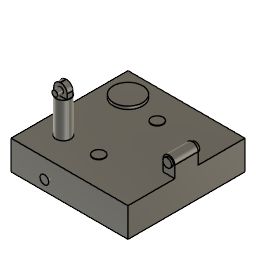
Soil Detector Rover (Autodesk Fusion 360 archive; units mm, degrees)
design "base"
part number: 2026-08-26-18-15-48-406
Autodesk Fusion 360 part; units mm, degrees
sketch "Sketch1" plane through (0, 0, 0) normal (0, 0, 1) x (1, 0, 0)
  line L0 (100, 100) -> (-100, 100)
  line L1 (-100, 100) -> (-100, -100)
  line L2 (-100, -100) -> (100, -100)
  line L3 (100, -100) -> (100, 100)
  line L4 (100, 100) -> (-100, -100) construction
  line L5 (-100, 100) -> (100, -100) construction
  dimension "d1" = 200
  dimension "d2" = 200
  constraint horizontal L0
  constraint perpendicular L0 L1
  constraint parallel L0 L2
  constraint parallel L1 L3
  constraint coincident L4 origin
  constraint coincident L5 origin
  measures "d1" distance of L0.end L1.end
  measures "d2" distance of L0.start L0.end
extrude "Extrude1" add sketch "Sketch1" along normal blind 50 makes body 1
sketch "Sketch2" plane through (0, 0, 50) normal (0, 0, 1) x (-1, 0, 0)
  line L0 (-100, 100) -> (-100, -100)
  line L1 (-100, -100) -> (100, -100)
  line L2 (100, -100) -> (100, 100)
  line L3 (100, 100) -> (-100, 100)
  circle A0 centre (60, 50.4709) radius 12.5
  dimension "d5" = 25
  dimension "d6" = 40
  measures "d5" diameter of A0
  measures "d6" distance of L2 A0.centre
extrude "Extrude2" add sketch "Sketch2" along normal blind 60 contours A0 bodies 1
sketch "Sketch3" plane through (0, 0, 110) normal (0, 0, 1) x (-1, 0, 0)
  circle A0 centre (60, 50.4709) radius 12.5
  line L0 (71.4564, 55.4709) -> (48.5436, 55.4709)
  line L1 (48.5436, 55.4709) -> (48.5436, 45.4709)
  line L2 (48.5436, 45.4709) -> (71.4564, 45.4709)
  line L3 (71.4564, 45.4709) -> (71.4564, 55.4709)
  line L4 (71.4564, 55.4709) -> (48.5436, 45.4709) construction
  line L5 (48.5436, 55.4709) -> (71.4564, 45.4709) construction
  circle A1 centre (60, 50.4709) radius 12.5
  point P0 (60, 50.4709)
  dimension "d10" = 10
  constraint horizontal L0
  constraint perpendicular L0 L1
  constraint parallel L0 L2
  constraint parallel L1 L3
  constraint coincident L4 P0
  constraint coincident L5 P0
  constraint coincident P0 A0.centre
  constraint coincident L1.end A1
  measures "d10" distance of L0.end L1.end
extrude "Extrude3" add sketch "Sketch3" along normal blind 20 contours L0 L1 L2 L3 bodies 1
fillet "Fillet1" radius 11.3 2 edges at (-71.4564, -50.4709, 130) (-48.5436, -50.4709, 130) on bodies 1
sketch "Sketch4" plane through (0, -55.4709, 0) normal (0, -1, 0) x (1, 0, 0)
  arc A0 (-48.5436, 118.7) -> (-59.8436, 130) centre (-59.8436, 118.7) ccw
  line L0 (-59.8436, 130) -> (-60.1564, 130)
  arc A1 (-60.1564, 130) -> (-71.4564, 118.7) centre (-60.1564, 118.7) ccw
  line L1 (-71.4564, 118.7) -> (-71.4564, 110)
  line L2 (-71.4564, 110) -> (-48.5436, 110)
  line L3 (-48.5436, 110) -> (-48.5436, 118.7)
  circle A2 centre (-59.8436, 118.7) radius 5
  dimension "d18" = 10
  constraint concentric A0 A2
  measures "d18" diameter of A2
extrude "Extrude4" add sketch "Sketch4" along normal blind 10 contours A2 bodies 1
sketch "Sketch5" plane through (0, 0, 50) normal (0, 0, 1) x (-1, 0, 0)
  circle A0 centre (60, 50.4709) radius 12.5
  line L0 (-100, 100) -> (-100, -100)
  line L1 (-100, -100) -> (100, -100)
  line L2 (100, -100) -> (100, 100)
  line L3 (100, 100) -> (-100, 100)
  line L4 (100, -60) -> (0, -60) construction
  line L5 (60, -100) -> (60, 0) construction
  circle A1 centre (60, -60) radius 25
  dimension "d21" = 50
  constraint coincident L2 L4.start
  constraint perpendicular L2 L4
  constraint coincident L1 L5.start
  constraint perpendicular L4 L5
  constraint coincident L4 A1.centre
  constraint coincident L5 A1.centre
  measures "d21" diameter of A1
extrude "Extrude5" add sketch "Sketch5" along normal blind 5 contours A1 bodies 1
sketch "Sketch6" plane through (0, -100, 0) normal (0, -1, 0) x (1, 0, 0)
  line L0 (-100, 0) -> (100, 0)
  line L1 (100, 0) -> (100, 50)
  line L2 (100, 50) -> (-100, 50)
  line L3 (-100, 50) -> (-100, 0)
  circle A0 centre (-40, 20) radius 7.5
  dimension "d24" = 15
  dimension "d25" = 60
  dimension "d26" = 20
  measures "d24" diameter of A0
  measures "d25" distance of L3 A0.centre
  measures "d26" distance of L0 A0.centre
extrude "Extrude6" add sketch "Sketch6" along normal blind 3 and the other way blind 203 separate body contours A0 makes body 2
sketch "Sketch7" plane through (0, 0, 50) normal (0, 0, 1) x (-1, 0, 0)
  circle A0 centre (60, -60) radius 25
  circle A1 centre (60, 50.4709) radius 12.5
  line L0 (-100, 100) -> (-100, -100)
  line L1 (-100, -100) -> (100, -100)
  line L2 (100, -100) -> (100, 100)
  line L3 (100, 100) -> (-100, 100)
  line L4 (-100, -20) -> (-80, -20)
  line L5 (-80, -20) -> (-80, 20)
  line L6 (-80, 20) -> (-100, 20)
  line L7 (-100, 20) -> (-100, -20)
  dimension "d31" = 20
  dimension "d32" = 40
  constraint horizontal L4
  constraint vertical L5
  constraint horizontal L6
  constraint vertical L7
  constraint coincident L0 L4.start
  measures "d31" distance of L4.start L4.end
  measures "d32" distance of L4.end L5.end
extrude "Extrude7" add sketch "Sketch7" along normal blind 30 contours L0 L4 L5 L6 L7 bodies 1
fillet "Fillet2" radius 10 2 edges at (100, 0, 80) (80, 0, 80) on bodies 1
sketch "Sketch8" plane through (0, -20, 0) normal (0, -1, 0) x (1, 0, 0)
  arc A0 (100, 70) -> (80, 70) centre (90, 70) ccw
  line L0 (80, 70) -> (80, 50)
  line L1 (80, 50) -> (100, 50)
  line L2 (100, 50) -> (100, 70)
  circle A1 centre (90, 70) radius 7.5
  dimension "d37" = 15
  constraint concentric A0 A1
  measures "d37" diameter of A1
extrude "Extrude8" add sketch "Sketch8" along normal blind 3 contours A1 bodies 1
sketch "Sketch9" plane through (0, 0, 50) normal (0, 0, 1) x (-1, 0, 0)
  line L0 (-80, -20) -> (-100, -20)
  line L1 (-100, -20) -> (-100, -100)
  line L2 (-100, -100) -> (100, -100)
  line L3 (100, -100) -> (100, 100)
  line L4 (100, 100) -> (-100, 100)
  line L5 (-100, 100) -> (-100, 20)
  line L6 (-100, 20) -> (-80, 20)
  line L7 (-80, 20) -> (-80, -20)
  circle A0 centre (60, -60) radius 25
  circle A1 centre (60, 50.4709) radius 12.5
  circle A2 centre (0, 50) radius 10
  circle A3 centre (0, -50) radius 10
  dimension "d40" = 20
  dimension "d41" = 20
  measures "d40" diameter of A2
  measures "d41" diameter of A3
extrude "Extrude9" add sketch "Sketch9" along normal blind 1 contours A2 | A3 bodies 1
sketch "Sketch10" plane through (0, 20, 0) normal (0, 1, 0) x (-1, 0, 0)
  arc A0 (-80, 70) -> (-100, 70) centre (-90, 70) ccw
  line L0 (-100, 70) -> (-100, 50)
  line L1 (-100, 50) -> (-80, 50)
  line L2 (-80, 50) -> (-80, 70)
  circle A1 centre (-90, 70) radius 7.5
  dimension "d44" = 15
  constraint concentric A0 A1
  measures "d44" diameter of A1
extrude "Extrude10" add sketch "Sketch10" along normal blind 5 contours A1 bodies 1
